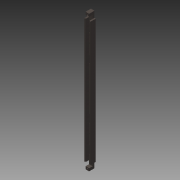
# Autodesk Inventor part: 13_1087_007
Saved by Autodesk Inventor 2014 SP1 (Build 180222100, 222)
## iProperties
Created: 2013-08-07
Part Number: 13_1087_007
Material: Allgemein
Document SubType Name: Modeling
Designer: vogel
Density: 1 g/cm^3
Appearance: Walnuss
Author: vogel
Autodesk Inventor part; units mm, degrees
ref_plane "YZ Plane" through (0, 0, 0) normal (1, 0, 0) x (0, 1, 0)
ref_plane "XZ Plane" through (0, 0, 0) normal (0, 1, 0) x (-1, 0, 0)
ref_plane "XY Plane" through (0, 0, 0) normal (0, 0, 1) x (1, 0, 0)
sketch "Skizze1" plane through (0, 0, 0) normal (0, 0, 1) x (1, 0, 0)
  line L0 (-9.8, 0) -> (9.8, 0) projected
  line L1 (0, -8.4) -> (0, 8.4) projected
  line L2 (-7, 6) -> (7, 6)
  line L3 (7, 6) -> (7, -6)
  line L4 (7, -6) -> (-7, -6)
  line L5 (-7, -6) -> (-7, 6)
  point P0 (0, 0)
  dimension "d0" = 14
  dimension "d1" = 12
  constraints: 8 end point, 2 parallel, 1 horizontal, 1 perpendicular, 2 other
  measures "d0" distance of L2.start L2.end
  measures "d1" distance of L4.end L2.start
extrude "Extrusion1" add sketch "Skizze1" along normal mid plane 308
sketch "Skizze2" plane through (-7, 6, 154) normal (0, 1, 0) x (1, 0, 0)
  line L0 (0, 308) -> (0, 0) projected
  line L1 (0, 308) -> (3, 308)
  line L2 (3, 308) -> (3, 294)
  line L3 (3, 294) -> (0, 294)
  line L4 (0, 294) -> (0, 308)
  line L5 (14, 308) -> (11, 308)
  line L6 (11, 308) -> (11, 294)
  line L7 (11, 294) -> (14, 294)
  line L8 (14, 294) -> (14, 308)
  line L9 (14, 0) -> (11, 0)
  line L10 (11, 0) -> (11, 14)
  line L11 (11, 14) -> (14, 14)
  line L12 (14, 14) -> (14, 0)
  line L13 (0, 0) -> (3, 0)
  line L14 (3, 0) -> (3, 14)
  line L15 (3, 14) -> (0, 14)
  line L16 (0, 14) -> (0, 0)
  point P0 (7, 154)
  dimension "d4" = 14
  dimension "d5" = 8
  dimension "d6" = 3
  dimension "d9" = 14
  dimension "d10" = 8
  dimension "d11" = 3
  constraints: 32 end point, 8 parallel, 4 horizontal, 4 perpendicular, 2 collinear
  measures "d4" distance of L5.end L6.end
  measures "d5" distance between parallel lines of L2 L6
  measures "d6" distance between parallel lines of L0 L2
  measures "d9" distance of L15.end L0.end
  measures "d10" distance between parallel lines of L10 L14
  measures "d11" distance between parallel lines of L0 L14
extrude "Extrusion2" cut sketch "Skizze2" against normal through all
sketch "Skizze3" plane through (-4, 6, 154) normal (0, 1, 0) x (1, 0, 0)
  line L0 (8, 0) -> (0, 0) projected
  line L1 (0, 308) -> (8, 308) projected
  line L2 (0, 308) -> (0, 294) projected
  point P0 (4, 154)
  point P1 (4, 304)
  point P2 (4, 4)
  dimension "d12" = 4
  dimension "d13" = 4
  dimension "d14" = 4
  constraints: 1 vertical alignment
  measures "d12" distance from line of point (4, 304) L1
  measures "d13" distance from line of L2 point (4, 304)
  measures "d14" distance from line of point (4, 4) L0
hole "Bohrung1" at (0, 6, -150) at (0, 6, 150) direction (0, -1, 0) diameter 3.4 end through all countersink diameter 6.9 countersink angle 90
sketch "Skizze4" plane through (-4, -6, -154) normal (0, -1, 0) x (1, 0, 0)
  circle A0 centre (4, 4) radius 1.7 projected
  circle A1 centre (4, 304) radius 1.7 projected
  line L0 (0, 294) -> (-3, 294) projected
  line L1 (-3, 294) -> (-3, 14) projected
  line L2 (-3, 14) -> (0, 14) projected
  line L3 (0, 14) -> (0, 0) projected
  line L4 (8, 0) -> (0, 0) projected
  line L5 (8, 0) -> (8, 14) projected
  line L6 (8, 14) -> (11, 14) projected
  line L7 (11, 294) -> (11, 14) projected
  line L8 (11, 294) -> (8, 294) projected
  line L9 (8, 294) -> (8, 308) projected
  line L10 (0, 308) -> (8, 308) projected
  line L11 (0, 308) -> (0, 294) projected
  line L12 (0, 6) -> (8, 6) projected
  line L13 (8, 302) -> (0, 302) projected
  line L14 (0, 302) -> (8, 302)
  line L15 (8, 302) -> (8, 6)
  line L16 (8, 6) -> (0, 6)
  line L17 (0, 6) -> (0, 302)
  point P0 (4, 154)
  constraints: 8 end point, 2 parallel, 1 horizontal, 1 perpendicular
extrude "Extrusion3" cut sketch "Skizze4" against normal blind 8 contours L11 L13 L9 L15 L5 L12 L3 L17
sketch "Skizze5" plane through (7, -6, -140) normal (0, -1, 0) x (1, 0, 0)
  line L0 (-3, 0) -> (0, 0) projected
  line L1 (-11, 0) -> (-11, 280) projected
  line L2 (-11, 280) -> (-14, 280) projected
  line L3 (-14, 280) -> (-14, 0) projected
  line L4 (-14, 0) -> (-11, 0) projected
  line L5 (-12.5, 280) -> (-1.5, 280)
  line L6 (-1.5, 280) -> (-1.5, 0)
  line L7 (-1.5, 0) -> (-12.5, 0)
  line L8 (-12.5, 0) -> (-12.5, 280)
  point P0 (-7, 140)
  constraints: 8 end point, 2 midpoint, 2 parallel, 1 horizontal, 1 perpendicular
extrude "Extrusion4" cut sketch "Skizze5" against normal blind 1 contours L7 L1 L5 L6 L0 | L4 L8 L2 L1
sketch "Skizze6" plane through (-4, 2, -154) normal (0, -1, 0) x (1, 0, 0)
  point P0 (4, 154)
  point P1 (4, 154)
  constraints: 1 coincident
hole "Bohrung2" at (0, 2, 0) direction (0, 1, 0) diameter 4.459 end through all thread size "M5x0.5" class "6H" standard "ISO Metric profile"
sketch "Skizze8" plane through (-4, 2, -154) normal (0, -1, 0) x (1, 0, 0)
  line L0 (0, 14) -> (0, 294) projected
  line L1 (4, 161.5) -> (4, 146.5)
  line L2 (-5.8, 154) -> (13.8, 154) projected
  line L3 (4, -61.6) -> (4, 369.6) projected
  point P0 (0, 167.3229)
  dimension "d42" = 15
  constraints: 2 coincident, 2 end point, 1 collinear, 1 parallel, 1 symmetric about line
  measures "d42" distance of point (4, 146.5) point (4, 161.5)
hole "Bohrung4" at (0, 2, 7.5) at (0, 2, -7.5) direction (0, 1, 0) diameter 1.567 end through all thread size "M2x0.4" class "6H" standard "ISO Metric profile"
sketch "Skizze9" plane through (-4, 6, 154) normal (0, 1, 0) x (1, 0, 0)
  line L0 (-5.8, 154) -> (13.8, 154) projected
  line L1 (4, 369.6) -> (4, -61.6) projected
  line L2 (6, 190) -> (6, 170)
  line L3 (2, 170) -> (2, 190)
  arc A0 (4, 168) -> (6, 170) centre (4, 170) ccw
  arc A1 (2, 170) -> (4, 168) centre (4, 170) ccw
  arc A2 (4, 192) -> (2, 190) centre (4, 190) ccw
  arc A3 (6, 190) -> (4, 192) centre (4, 190) ccw
  point P0 (6, 168)
  point P1 (6, 192)
  point P2 (2, 168)
  dimension "d50" = 4
  dimension "d52" = 24
  dimension "d53" = 2
  dimension "d54" = 14
  constraints: 8 point on circle, 4 centre point, 4 end point, 4 tangent, 3 equal radius, 3 point on line, 1 parallel, 1 vertical, 14 other
  measures "d50" distance of point (6, 168) point (2, 168)
  measures "d52" distance of point (6, 192) point (6, 168)
  measures "d53" radius of A0
  measures "d54" distance from line of A0.start L0
extrude "Extrusion5" cut sketch "Skizze9" against normal blind 3.5
mirror "Spiegeln1" about plane through (0, 0, 0) normal (0, 0, 1) of "Extrusion5"
sketch "Skizze10" plane through (-4, 2, -154) normal (0, -1, 0) x (1, 0, 0)
  circle A0 centre (4, 49.5) radius 1.2295 projected
  circle A1 centre (4, 49.5) radius 1.2295 projected
  circle A2 centre (4, 65.5) radius 1.2295 projected
  arc A3 (8, 106) -> (6, 108) centre (6, 106) ccw projected
  line L0 (11, 108) -> (6, 108) projected
  line L1 (11, 7) -> (11, 108) projected
  line L2 (11, 7) -> (6, 7) projected
  arc A4 (6, 7) -> (8, 9) centre (6, 9) ccw projected
  line L3 (8, 9) -> (8, 45) projected
  arc A5 (8, 45) -> (6, 47) centre (6, 45) ccw projected
  line L4 (6, 47) -> (2, 47) projected
  arc A6 (2, 47) -> (0, 45) centre (2, 45) ccw projected
  line L5 (0, 45) -> (0, 9) projected
  arc A7 (0, 9) -> (2, 7) centre (2, 9) ccw projected
  line L6 (2, 7) -> (-4, 7) projected
  line L7 (-4, 7) -> (-4, 108) projected
  line L8 (2, 108) -> (-4, 108) projected
  arc A8 (2, 108) -> (0, 106) centre (2, 106) ccw projected
  line L9 (0, 106) -> (0, 70) projected
  arc A9 (0, 70) -> (2, 68) centre (2, 70) ccw projected
  line L10 (2, 68) -> (6, 68) projected
  arc A10 (6, 68) -> (8, 70) centre (6, 70) ccw projected
  line L11 (8, 70) -> (8, 106) projected
  circle A11 centre (4, 65.5) radius 1.2295 projected
  circle A12 centre (4, 242.5) radius 1.2295 projected
  circle A13 centre (4, 258.5) radius 1.2295 projected
  constraints: 4 coincident
hole "Bohrung5" at (0, 2, 88.5) at (0, 2, 104.5) at (0, 2, -104.5) at (0, 2, -88.5) direction (0, 1, 0) diameter 3.4 end through all countersink diameter 6.9 countersink angle 90
sketch "Skizze11" plane through (-4, 2, -154) normal (0, -1, 0) x (1, 0, 0)
  line L0 (8, 106) -> (8, 70) projected
  line L1 (0, 106) -> (0, 70) projected
  circle A0 centre (4, 242.5) radius 1.2295 projected
  circle A1 centre (4, 258.5) radius 1.2295 projected
  arc A2 (8, 299) -> (6, 301) centre (6, 299) ccw projected
  line L2 (11, 301) -> (6, 301) projected
  line L3 (11, 200) -> (11, 301) projected
  line L4 (11, 200) -> (6, 200) projected
  arc A3 (6, 200) -> (8, 202) centre (6, 202) ccw projected
  line L5 (8, 202) -> (8, 238) projected
  arc A4 (8, 238) -> (6, 240) centre (6, 238) ccw projected
  line L6 (6, 240) -> (2, 240) projected
  arc A5 (2, 240) -> (0, 238) centre (2, 238) ccw projected
  line L7 (0, 238) -> (0, 202) projected
  arc A6 (0, 202) -> (2, 200) centre (2, 202) ccw projected
  line L8 (2, 200) -> (-4, 200) projected
  line L9 (-4, 200) -> (-4, 301) projected
  line L10 (2, 301) -> (-4, 301) projected
  arc A7 (2, 301) -> (0, 299) centre (2, 299) ccw projected
  line L11 (0, 299) -> (0, 263) projected
  arc A8 (0, 263) -> (2, 261) centre (2, 263) ccw projected
  line L12 (2, 261) -> (6, 261) projected
  arc A9 (6, 261) -> (8, 263) centre (6, 263) ccw projected
  line L13 (8, 263) -> (8, 299) projected
  circle A10 centre (4, 49.5) radius 1.2295 projected
  circle A11 centre (4, 65.5) radius 1.2295 projected
  arc A12 (8, 106) -> (6, 108) centre (6, 106) ccw projected
  line L14 (11, 108) -> (6, 108) projected
  line L15 (11, 7) -> (11, 108) projected
  line L16 (11, 7) -> (6, 7) projected
  arc A13 (6, 7) -> (8, 9) centre (6, 9) ccw projected
  line L17 (8, 9) -> (8, 45) projected
  arc A14 (8, 45) -> (6, 47) centre (6, 45) ccw projected
  line L18 (6, 47) -> (2, 47) projected
  arc A15 (2, 47) -> (0, 45) centre (2, 45) ccw projected
  line L19 (0, 45) -> (0, 9) projected
  arc A16 (0, 9) -> (2, 7) centre (2, 9) ccw projected
  line L20 (2, 7) -> (-4, 7) projected
  line L21 (-4, 7) -> (-4, 108) projected
  line L22 (2, 108) -> (-4, 108) projected
  arc A17 (2, 108) -> (0, 106) centre (2, 106) ccw projected
  line L23 (0, 106) -> (0, 70) projected
  arc A18 (0, 70) -> (2, 68) centre (2, 70) ccw projected
  line L24 (2, 68) -> (6, 68) projected
  arc A19 (6, 68) -> (8, 70) centre (6, 70) ccw projected
  line L25 (8, 70) -> (8, 106) projected
  line L26 (6, 106) -> (2, 106)
  line L27 (0, 104) -> (0, 88)
  line L28 (2, 86) -> (6, 86)
  line L29 (8, 88) -> (8, 104)
  line L30 (6, 45) -> (2, 45)
  line L31 (0, 43) -> (0, 27)
  line L32 (2, 25) -> (6, 25)
  line L33 (8, 27) -> (8, 43)
  line L34 (6, 202) -> (2, 202)
  line L35 (0, 204) -> (0, 220)
  line L36 (2, 222) -> (6, 222)
  line L37 (8, 220) -> (8, 204)
  line L38 (6, 263) -> (2, 263)
  line L39 (0, 265) -> (0, 281)
  line L40 (2, 283) -> (6, 283)
  line L41 (8, 281) -> (8, 265)
  arc A20 (8, 281) -> (6, 283) centre (6, 281) ccw
  arc A21 (6, 263) -> (8, 265) centre (6, 265) ccw
  arc A22 (0, 265) -> (2, 263) centre (2, 265) ccw
  arc A23 (2, 283) -> (0, 281) centre (2, 281) ccw
  arc A24 (2, 222) -> (0, 220) centre (2, 220) ccw
  arc A25 (0, 204) -> (2, 202) centre (2, 204) ccw
  arc A26 (6, 202) -> (8, 204) centre (6, 204) ccw
  arc A27 (8, 220) -> (6, 222) centre (6, 220) ccw
  arc A28 (8, 104) -> (6, 106) centre (6, 104) ccw
  arc A29 (0, 88) -> (2, 86) centre (2, 88) ccw
  arc A30 (6, 86) -> (8, 88) centre (6, 88) ccw
  arc A31 (2, 106) -> (0, 104) centre (2, 104) ccw
  arc A32 (2, 45) -> (0, 43) centre (2, 43) ccw
  arc A33 (0, 27) -> (2, 25) centre (2, 27) ccw
  arc A34 (6, 25) -> (8, 27) centre (6, 27) ccw
  arc A35 (8, 43) -> (6, 45) centre (6, 43) ccw
  point P0 (0, 86)
  point P1 (0, 25)
  point P2 (0, 222)
  point P3 (0, 283)
  dimension "d64" = 20
  dimension "d65" = 20
  dimension "d66" = 20
  dimension "d67" = 20
  dimension "d68" = 2
  constraints: 32 end point, 32 point on circle, 32 tangent, 20 point on line, 16 centre point, 15 equal radius, 8 parallel, 4 horizontal, 4 perpendicular
  measures "d64" distance between parallel lines of L26 L28
  measures "d65" distance between parallel lines of L30 L32
  measures "d66" distance between parallel lines of L38 L40
  measures "d67" distance from line of A3.centre L36
  measures "d68" radius of A20
extrude "Extrusion6" cut sketch "Skizze11" against normal through all contours L0 A30 L28 A29 L1 A31 L26 A28 | A34 L32 A33 L19 A32 L30 A35 L17 | L13 A21 L38 A22 L11 A23 L40 A20 | A26 L34 A25 L7 A24 L36 A27 L5
sketch "Skizze12" plane through (-4, 2, -154) normal (0, -1, 0) x (1, 0, 0)
  circle A0 centre (4, 56) radius 1.25 projected
  circle A1 centre (4, 252) radius 1.25 projected
  point P0 (4, 154)
  constraints: 2 coincident
hole "Bohrung6" at (0, 2, 98) at (0, 2, -98) direction (0, 1, 0) diameter 1.567 end through all thread size "M2x0.4" class "6H" standard "ISO Metric profile"
